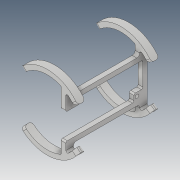
# Autodesk Inventor part: cameraMount3
Saved by Autodesk Inventor 2018 (Build 220112000, 112)
## iProperties
Created: 2020-04-09
Part Number: cameraMount3
Material: Generic
Document SubType Name: Modeling
Designer: anirudh
Density: 1 g/cm^3
Appearance: Default
Author: anirudh
Autodesk Inventor part; units mm, degrees
ref_plane "YZ Plane" through (0, 0, 0) normal (1, 0, 0) x (0, 1, 0)
ref_plane "XZ Plane" through (0, 0, 0) normal (0, 1, 0) x (-1, 0, 0)
ref_plane "XY Plane" through (0, 0, 0) normal (0, 0, 1) x (1, 0, 0)
sketch "Sketch1" plane through (0, 0, 0) normal (1, 0, 0) x (0, 1, 0)
  line L0 (17.5, 25.02) -> (22, 25.02)
  line L1 (22, 14.52) -> (22, -27.48)
  circle A0 centre (2.54, -23.48) radius 1.25
  line L2 (5, -21.48) -> (5, -27.48)
  line L3 (0, -21.48) -> (5, -21.48)
  arc A1 (20.3439, 15.1361) -> (18.21, 16.02) centre (19.46, 16.02) ccw
  line L4 (22, 14.52) -> (20.96, 14.52)
  line L5 (17.5, 16.02) -> (17.5, 25.02)
  line L6 (22, 25.02) -> (25.175, 25.02)
  line L7 (25.175, 25.02) -> (25.175, -30.48)
  line L8 (-3.175, -30.48) -> (-3.175, -21.48)
  line L9 (18.21, 16.02) -> (17.5, 16.02)
  line L10 (20.3439, 15.1361) -> (20.96, 14.52)
  line L11 (25.175, -30.48) -> (25.175, -27.48)
  line L12 (22, -27.48) -> (5, -27.48)
  line L13 (25.175, -30.48) -> (-3.175, -30.48)
  line L14 (-3.175, -30.48) -> (-3.175, 25.02)
  line L15 (-3.175, 25.02) -> (0, 25.02)
  line L16 (0, 25.02) -> (0, -21.48)
  constraints: 34 end point, 6 perpendicular, 4 horizontal, 2 centre point, 2 point on circle, 1 point on line, 1 vertical
extrude "Extrusion1" add sketch "Sketch1" against normal blind 3.175
sketch "Sketch2" plane through (0, -3.175, -30.48) normal (0, 0, -1) x (-1, 0, 0)
  line L0 (28.4154, 29.8904) -> (30.6605, 32.1355)
  line L1 (28.4154, -1.5404) -> (30.6605, -3.7855)
  line L2 (0, 28.35) -> (3.175, 28.35) projected
  line L3 (0, 28.35) -> (0, 32.414)
  line L4 (0, 28.35) -> (3.175, 28.35)
  line L5 (3.175, 28.35) -> (3.175, 34.2555)
  arc A0 (28.4154, 29.8904) -> (3.175, 34.2555) centre (12.7, 14.175) ccw
  line L6 (0, 0) -> (0, -4.064)
  line L7 (0, 0) -> (3.175, 0) projected
  line L8 (0, 0) -> (3.175, 0)
  line L9 (3.175, 0) -> (3.175, -5.9055)
  arc A1 (3.175, -5.9055) -> (28.4154, -1.5404) centre (12.7, 14.175) ccw
  line L10 (-5.5057, 26.9227) -> (-8.1065, 28.7438)
  line L11 (-5.5057, 1.4273) -> (-8.1065, -0.3938)
  arc A2 (30.6605, 32.1355) -> (-8.1065, 28.7438) centre (12.7, 14.175) ccw
  arc A3 (-8.1065, -0.3938) -> (30.6605, -3.7855) centre (12.7, 14.175) ccw
  arc A4 (0, 32.414) -> (-5.5057, 26.9227) centre (12.7, 14.175) ccw
  arc A5 (-5.5057, 1.4273) -> (0, -4.064) centre (12.7, 14.175) ccw
  constraints: 20 end point, 12 point on circle, 6 centre point, 2 horizontal, 2 perpendicular, 2 vertical, 1 coincident
extrude "Extrusion2" add sketch "Sketch2" against normal blind 5.08
sketch "Sketch3" plane through (0, 17.5, 25.02) normal (0, 0, 1) x (1, 0, 0)
  line L0 (0, 7.675) -> (-3.175, 7.675) projected
  arc A0 (-3.175, 13.5805) -> (-28.4154, 9.2154) centre (-12.7, -6.5) ccw projected
  line L1 (-3.175, 7.675) -> (-3.175, 13.5805)
  line L2 (-3.175, 7.675) -> (0, 7.675)
  arc A1 (5.5057, 6.2477) -> (0, 11.739) centre (-12.7, -6.5) ccw projected
  line L3 (0, 7.675) -> (0, 11.739)
  line L4 (0, -24.739) -> (0, 11.739) projected
  line L5 (-3.175, -20.675) -> (-3.175, -17.5) projected
  arc A2 (-28.4154, -22.2154) -> (-3.175, -26.5805) centre (-12.7, -6.5) ccw projected
  line L6 (-3.175, -20.675) -> (0, -20.675) projected
  line L7 (-3.175, -26.5805) -> (-3.175, 13.5805) projected
  line L8 (-3.175, -20.675) -> (-3.175, -26.5805)
  line L9 (-3.175, -20.675) -> (0, -20.675)
  line L10 (0, -17.5) -> (0, -20.675) projected
  line L11 (0, -20.675) -> (0, -24.739)
  line L12 (5.5057, 6.2477) -> (8.1065, 8.0688) projected
  line L13 (-28.4154, 9.2154) -> (-30.6605, 11.4605) projected
  line L14 (-28.4154, 9.2154) -> (-30.6605, 11.4605)
  line L15 (-30.6605, -24.4605) -> (-28.4154, -22.2154) projected
  line L16 (-28.4154, -22.2154) -> (-30.6605, -24.4605)
  line L17 (5.5057, -19.2477) -> (8.1065, -21.0688) projected
  arc A3 (-30.6605, -24.4605) -> (8.1065, -21.0688) centre (-12.7, -6.5) ccw
  arc A4 (8.1065, 8.0688) -> (-30.6605, 11.4605) centre (-12.7, -6.5) ccw
  line L18 (5.5057, 6.2477) -> (8.1065, 8.0688)
  line L19 (5.5057, -19.2477) -> (8.1065, -21.0688)
  arc A5 (-28.4154, -22.2154) -> (-3.175, -26.5805) centre (-12.7, -6.5) ccw
  arc A6 (0, -24.739) -> (5.5057, -19.2477) centre (-12.7, -6.5) ccw
  arc A7 (5.5057, 6.2477) -> (0, 11.739) centre (-12.7, -6.5) ccw
  arc A8 (-3.175, 13.5805) -> (-28.4154, 9.2154) centre (-12.7, -6.5) ccw
  constraints: 21 end point, 14 point on circle, 6 centre point, 5 collinear, 2 coincident, 2 vertical, 1 horizontal, 1 perpendicular, 1 point on line
extrude "Extrusion3" add sketch "Sketch3" against normal blind 5.08 contours L0 L1 A0 L13 A4 L12 A1 L3 | L4 A6 L17 A3 L15 A2 L7 L6
fillet "Fillet1" radius 1 7 edges at (-1.5875, 0, -21.48) (-1.5875, 5, -21.48) (-1.5875, 5, -27.48) (-1.5875, 22, -27.48) (-1.5875, 0, 25.02) (-1.5875, 17.5, 25.02) (-1.5875, 22, 14.52)
fillet "Fillet2" radius 2 16 edges at (6.8061, 24.6583, 25.02) (6.8061, 24.6583, 19.94) (-29.538, 27.838, 25.02) (-29.538, 27.838, 19.94) (6.8061, -2.6583, 25.02) (6.8061, -2.6583, 19.94) (6.8061, -2.6583, -25.4) (6.8061, -2.6583, -30.48) (6.8061, 24.6583, -25.4) (6.8061, 24.6583, -30.48) (-29.538, -5.838, -25.4) (-29.538, -5.838, -30.48) (-29.538, 27.838, -25.4) (-29.538, 27.838, -30.48) (-29.538, -5.838, 25.02) (-29.538, -5.838, 19.94)
fillet "Fillet3" radius 2 4 edges at (-1.5875, -3.175, -25.4) (-1.5875, 25.175, -25.4) (-1.5875, -3.175, 19.94) (-1.5875, 25.175, 19.94)
fillet "Fillet4" radius 1 8 edges at (0, -7.239, -27.94) (0, -7.239, 22.48) (-3.175, -9.0805, 22.48) (-3.175, -9.0805, -27.94) (0, 29.239, 22.48) (-3.175, 31.0805, 22.48) (0, 29.239, -27.94) (-3.175, 31.0805, -27.94)
body "Solid1"
